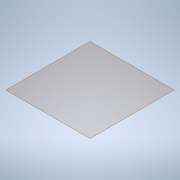
# Autodesk Inventor part: ceiling
Saved by Autodesk Inventor 2020.2 (Build 242310000, 310)
## iProperties
Created: 2020-01-09
Part Number: ceiling
Material: Polycarbonate, Smoke
Document SubType Name: Modeling
Designer: steele
Density: 1.2 g/cm^3
Appearance: Polycarbonate - Smoked
Author: steele
Autodesk Inventor part; units mm, degrees
ref_plane "YZ Plane" through (0, 0, 0) normal (1, 0, 0) x (0, 1, 0)
ref_plane "XZ Plane" through (0, 0, 0) normal (0, 1, 0) x (-1, 0, 0)
ref_plane "XY Plane" through (0, 0, 0) normal (0, 0, 1) x (1, 0, 0)
sketch "Sketch1" plane through (0, 0, 0) normal (0, 1, 0) x (-1, 0, 0)
  line L0 (508, 508) -> (-508, 508)
  line L1 (-508, 508) -> (-508, -508)
  line L2 (-508, -508) -> (508, -508)
  line L3 (508, -508) -> (508, 508)
  line L4 (508, 508) -> (-508, -508) construction
  line L5 (-508, 508) -> (508, -508) construction
  point P0 (0, 0)
  dimension "d0" = 1016
  dimension "d1" = 1016
  constraints: 12 end point, 2 midpoint, 2 parallel, 1 horizontal, 1 perpendicular
  measures "d0" distance of L0.start L0.end
  measures "d1" distance of L1.end L0.end
extrude "Extrusion1" add sketch "Sketch1" along normal blind 0.254
body "Solid1"
